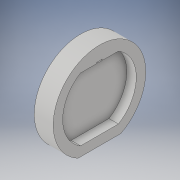
# Autodesk Inventor part: end cap
Saved by Autodesk Inventor 2017 (Build 210142000, 142)
## iProperties
Created: 2018-03-04
Part Number: end cap
Material: Generic
Document SubType Name: Modeling
Designer: Braxton
Density: 1 g/cm^3
Appearance: Default
Author: Braxton
Autodesk Inventor part; units mm, degrees
ref_plane "YZ Plane" through (0, 0, 0) normal (1, 0, 0) x (0, 1, 0)
ref_plane "XZ Plane" through (0, 0, 0) normal (0, 1, 0) x (-1, 0, 0)
ref_plane "XY Plane" through (0, 0, 0) normal (0, 0, 1) x (1, 0, 0)
sketch "Sketch1" plane through (0, 0, 0) normal (1, 0, 0) x (0, 1, 0)
  line L0 (-84.6667, -50.8) -> (-84.6667, 50.8)
  arc A0 (-110.0667, -57.4059) -> (-110.0667, 57.4059) centre (0, 0) ccw
  arc A1 (-84.6667, -50.8) -> (84.6667, -50.8) centre (0, 0) ccw
  arc A2 (84.6853, 50.7689) -> (-84.6667, 50.8) centre (0, 0) ccw
  line L1 (-110.0667, 57.4059) -> (-110.0667, -57.4059)
  line L2 (84.6853, 9.0287) -> (84.6667, -8.9655) construction
  arc A3 (86.254, -7.4006) -> (84.6667, -8.9655) centre (86.254, -8.9881) ccw
  arc A4 (84.6853, 9.0287) -> (86.2694, 7.4605) centre (86.2727, 9.048) ccw
  line L3 (84.6667, 0.0316) -> (87.8417, 0.0283) construction
  line L4 (87.8417, 7.4605) -> (86.2694, 7.4605)
  line L5 (84.6667, -50.8) -> (84.6667, -8.9655)
  line L6 (84.6853, 9.0287) -> (84.6853, 50.7689)
  line L7 (84.6259, -4.0844) -> (84.6259, 0)
  line L8 (85.3112, -5.7079) -> (86.8916, -4.0844) construction
  arc A5 (87.8417, -6.35) -> (84.6259, -3.1747) centre (84.6667, -6.3494) ccw construction
  line L9 (87.8417, -6.35) -> (86.8724, -6.35)
  arc A6 (84.6259, -4.0844) -> (86.8724, -6.35) centre (86.8916, -4.0844) ccw
  line L10 (84.6259, 4.0844) -> (84.6259, 0)
  line L11 (85.3112, 5.7079) -> (86.8916, 4.0844) construction
  line L12 (87.8417, 6.35) -> (86.8724, 6.35)
  arc A7 (84.6259, 3.1747) -> (87.8417, 6.35) centre (84.6667, 6.3494) ccw construction
  arc A8 (86.8724, 6.35) -> (84.6259, 4.0844) centre (86.8916, 4.0844) ccw
  line L13 (84.6259, 0) -> (87.8417, 0) construction
  line L14 (87.8417, 7.4605) -> (87.8417, 6.35)
  line L15 (87.8417, 6.35) -> (87.8417, 0)
  line L16 (87.8417, 0) -> (87.8417, -6.35)
  line L17 (87.8417, -6.35) -> (87.8417, -7.4006)
  line L18 (87.8417, -7.4006) -> (86.254, -7.4006)
  point P0 (87.8079, -3.1429)
  point P1 (87.8079, 3.1429)
  point P2 (86.9731, -7.378)
  dimension "d13" = 101.6
  dimension "d18" = 25.4
  dimension "d25" = 1.5875
  dimension "d32" = 6.35
  dimension "d33" = 3.175
  dimension "d34" = 2.2657
  dimension "d35" = 2.2466
  dimension "d36" = 3.2158
  constraints: 38 end point, 22 point on circle, 11 symmetric about line, 9 centre point, 4 coincident, 4 vertical, 2 collinear, 2 horizontal, 2 parallel, 2 perpendicular, 2 point on line, 1 tangent, 3 other
  measures "d13" distance of L0.start L0.end
  measures "d18" distance between parallel lines of L0 L1
  measures "d25" radius of A3
  measures "d32" distance of L13.end L12.start
  measures "d33" distance of L12.start point (84.667, 6.349)
  measures "d34" radius of A8
  measures "d35" horizontal distance of L10.start L12.end
  measures "d36" distance of L10.end L13.end
extrude "connection" add sketch "Sketch1" along normal blind 25.4
extrude "light\\" add sketch "Sketch1" along normal up to surface (25.4 mm away) separate body contours L9 A6 L7 L10 A8 L12 L15 L16
sketch "Sketch5" plane through (0, 0, 0) normal (-1, 0, 0) x (0, 0, -1)
  arc A0 (-57.4059, 110.0667) -> (57.4059, 110.0667) centre (0, 0) ccw
  line L0 (-57.4059, 110.0667) -> (57.4059, 110.0667) projected
  line L1 (-57.4059, 110.0667) -> (57.4059, 110.0667)
  constraints: 2 end point, 2 point on circle, 1 centre point, 1 coincident, 1 collinear
extrude "end cap" add sketch "Sketch5" along normal blind 25.4 bodies 1
body "Solid2"
body "Solid3"
